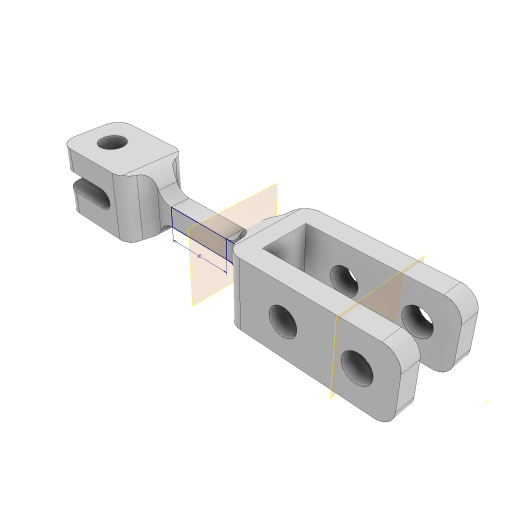
# Autodesk Inventor part: Acoplador
Saved by Autodesk Inventor 2023.5 (Build 275446020, 446B)
## iProperties
Created: 2025-07-10
Part Number: Acoplador
Material: Genérico
Document SubType Name: Modeling
Designer: jaime
Density: 1 g/cm^3
Appearance: Valor por defecto
Author: jaime
Autodesk Inventor part; units mm, degrees
ref_plane "YZ Plane" through (0, 0, 0) normal (1, 0, 0) x (0, 1, 0)
ref_plane "XZ Plane" through (0, 0, 0) normal (0, 1, 0) x (-1, 0, 0)
ref_plane "XY Plane" through (0, 0, 0) normal (0, 0, 1) x (1, 0, 0)
sketch "Boceto1" plane through (0, 0, 0) normal (0, 0, 1) x (1, 0, 0)
  circle A0 centre (0, 0) radius 2
  line L0 (0, 0) -> (10, 0)
  circle A1 centre (10, 0) radius 2
  line L1 (2, 0) -> (8, 0)
  line L2 (2, 0) -> (8, 0)
  line L3 (-5, -5) -> (15, -5)
  line L4 (15, -5) -> (15, 5)
  line L5 (15, 5) -> (-5, 5)
  line L6 (-5, -5) -> (15, 5) construction
  line L7 (15, -5) -> (-5, 5) construction
  line L8 (-5, 5) -> (-9, 5)
  line L9 (-9, 5) -> (-9, -5)
  line L10 (-9, -5) -> (-5, -5)
  point P0 (5, 0)
  dimension "d0" = 4
  dimension "d1" = 10
  dimension "d2" = 20
  dimension "d3" = 10
  dimension "d7" = 4
  constraints: 22 end point, 3 horizontal, 3 midpoint, 3 perpendicular, 2 coincident, 2 horizontal alignment, 2 point on line, 1 collinear, 1 parallel, 4 other
  measures "d1" distance of L0.start L0.end
  measures "d2" distance of L5.end L4.end
  measures "d3" distance of L4.end L3.end
  measures "d7" distance of L5.end L8.end
extrude "Extrusión1" add sketch "Boceto1" along normal blind 13
sketch "Boceto2" plane through (15, -5, 0) normal (1, 0, 0) x (0, 0, -1)
  line L0 (0, 10) -> (-13, 10) projected
  line L1 (-10, 0) -> (-3, 0)
  line L2 (-3, 0) -> (-3, 10)
  line L3 (-3, 10) -> (-10, 10)
  line L4 (-10, 10) -> (-10, 0)
  line L5 (-10, 0) -> (-3, 10) construction
  line L6 (-3, 0) -> (-10, 10) construction
  point P0 (0, 5)
  point P1 (-6.5, 5)
  dimension "d6" = 7
  constraints: 12 end point, 2 midpoint, 2 parallel, 1 horizontal, 1 perpendicular, 1 point on line
  measures "d6" distance of L3.end L2.end
extrude "Extrusión2" cut sketch "Boceto2" against normal blind 21
sketch "Boceto3" plane through (-9, -5, 0) normal (-1, 0, 0) x (0, 0, 1)
  line L0 (0, 0) -> (13, 0) projected
  line L1 (8, 10) -> (5, 10)
  line L2 (5, 10) -> (5, 0)
  line L3 (5, 0) -> (8, 0)
  line L4 (8, 0) -> (8, 10)
  line L5 (8, 10) -> (5, 0) construction
  line L6 (5, 10) -> (8, 0) construction
  point P0 (0, 5)
  point P1 (6.5, 5)
  dimension "d10" = 3
  constraints: 12 end point, 2 midpoint, 2 parallel, 1 horizontal, 1 perpendicular, 1 point on line
  measures "d10" distance of L3.end L2.end
extrude "Extrusión3" add sketch "Boceto3" along normal blind 55
sketch "Boceto4" plane through (-9, -5, 8) normal (0, 0, 1) x (1, 0, 0)
  line L0 (0, 10) -> (0, 0) projected
  line L1 (0, 5) -> (-48, 5)
  line L2 (-55, 10) -> (-55, 0) projected
  line L3 (-41, 3.5) -> (-55, 3.5)
  line L4 (-55, 3.5) -> (-55, 6.5)
  line L5 (-55, 6.5) -> (-41, 6.5)
  line L6 (-41, 6.5) -> (-41, 3.5)
  line L7 (-41, 3.5) -> (-55, 6.5) construction
  line L8 (-55, 3.5) -> (-41, 6.5) construction
  line L9 (-41, 3.5) -> (-41, 0)
  line L10 (0, 0) -> (-55, 0) projected
  line L11 (0, 10) -> (-55, 10) projected
  line L12 (-41, 6.5) -> (-55, 6.5)
  line L13 (-55, 6.5) -> (-55, 10)
  line L14 (-55, 10) -> (-41, 10)
  line L15 (-41, 10) -> (-41, 6.5)
  line L16 (-55, 3.5) -> (-41, 3.5)
  line L17 (-41, 3.5) -> (-41, 0)
  line L18 (-41, 0) -> (-55, 0)
  line L19 (-55, 0) -> (-55, 3.5)
  point P0 (9, 5)
  dimension "d13" = 48
  dimension "d14" = 3
  constraints: 32 end point, 6 parallel, 4 horizontal, 3 midpoint, 3 perpendicular, 2 point on line, 1 vertical
  measures "d13" distance of L1.start L1.end
  measures "d14" distance of L3.end L4.end
extrude "Extrusión4" cut sketch "Boceto4" against normal blind 55 contours L15 L5 L2 L11 | L10 L2 L3 L9
sketch "Boceto5" plane through (-64, 1.5, 8) normal (0, 1, 0) x (1, 0, 0)
  circle A0 centre (7, 1.5) radius 2
  line L0 (14, 6.5) -> (0, 6.5)
  line L1 (0, 6.5) -> (0, -3.5)
  line L2 (0, -3.5) -> (14, -3.5)
  line L3 (14, -3.5) -> (14, 6.5)
  line L4 (14, 6.5) -> (0, -3.5) construction
  line L5 (0, 6.5) -> (14, -3.5) construction
  point P0 (64, 8)
  dimension "d18" = 4
  dimension "d20" = 10
  constraints: 12 end point, 2 midpoint, 2 parallel, 1 centre point, 1 horizontal, 1 perpendicular
  measures "d18" diameter of A0
  measures "d20" distance of L1.end L0.end
extrude "Extrusión5" add sketch "Boceto5" against normal blind 3
sketch "Boceto6" plane through (-64, 1.5, 1.5) normal (0, 1, 0) x (1, 0, 0)
  arc A0 (8.3229, -3.5) -> (5.6771, -3.5) centre (7, -5) ccw projected
  circle A1 centre (7, -5) radius 2
  point P0 (64, 1.5)
  point P1 (5.6771, -3.5)
  point P2 (8.3229, -3.5)
  constraints: 1 centre point, 1 coincident
extrude "Extrusión6" cut sketch "Boceto6" against normal blind 3
sketch "Boceto7" plane through (-9, 5, 0) normal (0, 1, 0) x (1, 0, 0)
  line L0 (-41, -8) -> (-41, -11.5) projected
  line L1 (-41, -11.5) -> (-41, -10)
  line L2 (-39, -8) -> (-34.5905, -8)
  arc A0 (-39, -8) -> (-41, -10) centre (-39, -10) ccw
  line L3 (-41, -1.5) -> (-41, -5) projected
  line L4 (-38.5, -5) -> (-34.5905, -5)
  line L5 (0, -5) -> (-41, -5) projected
  line L6 (-41, -2.5) -> (-41, -1.5)
  arc A1 (-41, -2.5) -> (-38.5, -5) centre (-38.5, -2.5) ccw
  line L7 (-41, -2.5) -> (-41, -10)
  line L8 (-34.5905, -5) -> (-34.5905, -8)
  line L9 (0, -8) -> (-41, -8) projected
  point P0 (9, 0)
  point P1 (-38.5, -5)
  dimension "d25" = 2
  dimension "d26" = 2.5
  constraints: 12 end point, 5 point on line, 5 tangent, 4 point on circle, 3 perpendicular, 2 centre point, 1 collinear, 1 vertical
  measures "d25" radius of A0
  measures "d26" radius of A1
extrude "Extrusión7" add sketch "Boceto7" against normal blind 10 contours L9 A0 L0 | L3 A1 L5
sketch "Boceto8" plane through (-64, 1.5, 11.5) normal (0, 0, 1) x (1, 0, 0)
  line L0 (14, 3.5) -> (14, 0) projected
  line L1 (14, 3.5) -> (14, 3.5)
  line L2 (10.5, 0) -> (10.0047, 0)
  line L3 (0, 0) -> (14, 0) projected
  line L4 (0, -3) -> (14, -3) projected
  line L5 (10.0047, -3) -> (10.5, -3)
  line L6 (14, -3) -> (14, -6.5) projected
  line L7 (14, -6.5) -> (14, -6.5)
  line L8 (10.0047, -3) -> (10.0047, 0)
  line L9 (14, 2.5) -> (14, 3.5)
  arc A0 (14, -6.5) -> (10.5, -3) centre (10.5, -6.5) ccw
  arc A1 (10.5, 0) -> (14, 3.5) centre (10.5, 3.5) ccw
  line L10 (14, 2.5) -> (14, -6.5)
  point P0 (64, -1.5)
  point P1 (10.5, -3)
  dimension "d31" = 3.5
  dimension "d32" = 3.5
  constraints: 14 end point, 7 point on line, 4 point on circle, 4 tangent, 2 centre point, 2 collinear, 2 vertical, 1 perpendicular
  measures "d31" radius of A0
  measures "d32" radius of A1
extrude "Extrusión8" add sketch "Boceto8" against normal blind 10
sketch "Boceto9" plane through (-64, 1.5, 11.5) normal (0, 1, 0) x (1, 0, 0)
  line L0 (14, 0) -> (10.5, 0) projected
  line L1 (0, 10) -> (14, 10)
  line L2 (14, 10) -> (14, 0)
  line L3 (14, 0) -> (0, 0)
  line L4 (0, 0) -> (0, 10)
  circle A0 centre (7, 5) radius 2 projected
  circle A1 centre (7, 5) radius 2
  point P0 (64, 11.5)
  constraints: 8 end point, 2 parallel, 1 centre point, 1 coincident, 1 horizontal, 1 perpendicular
extrude "Extrusión9" add sketch "Boceto9" along normal blind 3.5
sketch "Boceto10" plane through (-64, -1.5, 1.5) normal (0, -1, 0) x (1, 0, 0)
  circle A0 centre (7, 5) radius 2 projected
  circle A1 centre (7, 5) radius 2
  line L0 (0, 10) -> (0, 0) projected
  line L1 (14, 0) -> (10.5, 0) projected
  line L2 (0, 10) -> (14, 10)
  line L3 (14, 10) -> (14, 0)
  line L4 (14, 0) -> (0, 0)
  line L5 (0, 0) -> (0, 10)
  point P0 (64, -1.5)
  constraints: 8 end point, 2 parallel, 1 centre point, 1 coincident, 1 horizontal, 1 perpendicular
extrude "Extrusión10" add sketch "Boceto10" along normal blind 3.5
sketch "Boceto11" plane through (-64, -5, 0) normal (-1, 0, 0) x (0, 0, 1)
  line L0 (11.5, 0) -> (11.5, 10) projected
  line L1 (1.5, 3.5) -> (11.5, 3.5)
  line L2 (11.5, 3.5) -> (11.5, 6.5)
  line L3 (11.5, 6.5) -> (1.5, 6.5)
  line L4 (1.5, 6.5) -> (1.5, 3.5)
  line L5 (1.5, 3.5) -> (11.5, 6.5) construction
  line L6 (11.5, 3.5) -> (1.5, 6.5) construction
  point P0 (0, 5)
  point P1 (6.5, 5)
  dimension "d39" = 3
  constraints: 12 end point, 2 midpoint, 2 parallel, 1 horizontal, 1 perpendicular, 1 point on line
  measures "d39" distance of L2.end L1.end
extrude "Extrusión11" cut sketch "Boceto11" against normal blind 11
fillet "Empalme1" radius 2.5 1 edges at (-50, 0, 1.5)
fillet "Empalme2" radius 2.5 1 edges at (-50, 0, 11.5)
fillet "Empalme3" radius 2.5 1 edges at (-9, 0, 5)
fillet "Empalme4" radius 2.5 1 edges at (-9, 0, 0)
fillet "Empalme5" radius 2.5 1 edges at (-9, 0, 8)
fillet "Empalme6" radius 2.5 1 edges at (-9, 0, 13)
sketch "Boceto12" plane through (-48, -5, 8) normal (0, 0, 1) x (1, 0, 0)
  line L0 (36.5, 10) -> (0, 10) projected
  line L1 (36.5, 10) -> (36.5, 0) projected
  line L2 (0, 10) -> (36.5, 10)
  line L3 (36.5, 10) -> (36.5, 9)
  line L4 (36.5, 0) -> (0, 0)
  line L5 (0, 9) -> (0, 10)
  line L6 (2.5, 3.5) -> (34, 3.5)
  line L7 (36.5, 3.5) -> (36.5, 6.5)
  line L8 (34, 6.5) -> (2.5, 6.5)
  line L9 (0, 6.5) -> (0, 3.5)
  line L10 (0, 3.5) -> (36.5, 6.5) construction
  line L11 (36.5, 3.5) -> (0, 6.5) construction
  arc A0 (0, 9) -> (2.5, 6.5) centre (2.5, 9) ccw
  arc A1 (34, 6.5) -> (36.5, 9) centre (34, 9) ccw
  line L12 (0, 0) -> (0, 10) projected
  line L13 (0, 1) -> (0, 0)
  line L14 (0, 0) -> (36.5, 0)
  arc A2 (2.5, 3.5) -> (0, 1) centre (2.5, 1) ccw
  line L15 (36.5, 1) -> (36.5, 0)
  arc A3 (36.5, 1) -> (34, 3.5) centre (34, 1) ccw
  line L16 (-4.3875, 10) -> (-4.3875, 0) projected
  line L17 (-4.3875, 6.5) -> (2.5, 6.5)
  line L18 (-4.3875, 10) -> (-4.3875, 6.5)
  point P0 (48, 5)
  point P1 (18.25, 5)
  dimension "d48" = 3
  dimension "d49" = 2.5
  dimension "d50" = 2.5
  dimension "d51" = 2.5
  dimension "d52" = 2.5
  constraints: 30 end point, 10 point on line, 8 point on circle, 8 tangent, 4 centre point, 4 parallel, 4 perpendicular, 2 collinear, 2 horizontal, 2 midpoint, 1 vertical
  measures "d48" distance of L7.end L7.start
  measures "d49" radius of A0
  measures "d50" radius of A1
  measures "d51" radius of A2
  measures "d52" radius of A3
extrude "Extrusión12" cut sketch "Boceto12" against normal blind 11 contours L1 A1 L8 A0 L5 L0 | L1 L4 L12 A2 L6 A3
fillet "Empalme7" radius 3.5 1 edges at (-11.5, 5, 6.5)
fillet "Empalme8" radius 3.5 1 edges at (-11.5, -5, 6.5)
fillet "Empalme9" radius 3.5 1 edges at (-48, 5, 6.4747)
fillet "Empalme10" radius 3.5 1 edges at (-48, -5, 6.4747)
fillet "Empalme11" radius 2.5 4 edges at (-64, 3.25, 11.5) (-64, -3.25, 11.5) (-64, 3.25, 1.5) (-64, -3.25, 1.5)
sketch "Boceto15" plane through (-50.9544, 5, 11.0485) normal (0, 1, 0) x (1, 0, 0)
  line L0 (-2.0456, 9.5485) -> (-2.0456, -0.4515) projected
  line L1 (-10.5456, 9.5485) -> (-2.0456, 9.5485) projected
  line L2 (-2.0456, -0.4515) -> (-8.0338, -0.4515)
  line L3 (-8.0338, -0.4515) -> (-8.0338, 9.5485)
  line L4 (-8.0338, 9.5485) -> (-2.0456, 9.5485)
  line L5 (-2.0456, 9.5485) -> (-2.0456, -0.4515)
  point P0 (50.9544, 11.0485)
  constraints: 8 end point, 2 parallel, 1 horizontal, 1 perpendicular, 1 point on line
extrude "Extrusión13" add sketch "Boceto15" against normal blind 10
sketch "Boceto16" plane through (-50.9544, 5, 11.0485) normal (0, 1, 0) x (1, 0, 0)
  line L0 (-13.0456, 7.0485) -> (-13.0456, 2.0485) projected
  line L1 (-13.0456, 4.5485) -> (-8.0456, 4.5485)
  circle A0 centre (-8.0456, 4.5485) radius 2
  point P0 (50.9544, 11.0485)
  dimension "d65" = 5
  dimension "d66" = 4
  constraints: 2 end point, 1 centre point, 1 coincident, 1 horizontal, 1 midpoint
  measures "d65" distance of L1.start L1.end
  measures "d66" diameter of A0
extrude "Extrusión14" cut sketch "Boceto16" against normal blind 10
sketch "Boceto17" plane through (-52.3875, -5, 11.5) normal (0, 0, 1) x (1, 0, 0)
  line L0 (-6.6007, 6.5) -> (-6.6007, 3.5) projected
  line L1 (-6.6007, 6.5) -> (-3.1007, 6.5)
  line L2 (-3.1007, 6.5) -> (-3.1007, 3.5)
  line L3 (-3.1007, 3.5) -> (-6.6007, 3.5)
  line L4 (-6.6007, 3.5) -> (-6.6007, 6.5)
  point P0 (52.3875, 5)
  dimension "d69" = 3.5
  dimension "d70" = 3
  constraints: 8 end point, 2 parallel, 1 horizontal, 1 perpendicular
  measures "d69" distance of L2.end L3.end
  measures "d70" distance of L1.end L2.end
extrude "Extrusión15" cut sketch "Boceto17" against normal blind 10
fillet "Empalme12" radius 2.5 4 edges at (15, 5, 11.5) (15, 5, 1.5) (15, -5, 1.5) (15, -5, 11.5)
sketch "Boceto18" plane through (-45.5, -1.5, 8) normal (0, 0, 1) x (1, 0, 0)
  line L0 (0, 3) -> (31.5, 3)
  line L1 (31.5, 3) -> (31.5, 0)
  line L2 (31.5, 0) -> (0, 0)
  line L3 (0, 0) -> (0, 3)
  line L4 (0, 3) -> (31.5, 3) projected
  line L5 (31.5, 0) -> (0, 0) projected
  line L6 (0, 3) -> (10, 3)
  line L7 (10, 3) -> (10, 0)
  line L8 (10, 0) -> (0, 0)
  line L9 (0, 0) -> (0, 3)
  point P0 (45.5, 1.5)
  dimension "d74" = 10
  constraints: 16 end point, 4 parallel, 2 horizontal, 2 perpendicular, 1 point on line
  measures "d74" distance of L7.end L8.end
ref_plane "Plano de trabajo1" through (-35.5, 1.5, 8) normal (1, 0, 0) x (0, -1, 0)
ref_plane "Plano de trabajo2" through (-14, 1.5, 8) normal (1, 0, 0) x (0, -1, 0)
split body "Dividir1" result two bodies by plane through (-35.5, 1.5, 8) normal (1, 0, 0) first body at (2.0803, 3.9951, 12.5)
split "Dividir2" plane through (-14, 1.5, 8) removes the side toward (-1, 0, 0) bodies 2
move or copy body "Desplazar cuerpo1" bodies to move or copy 2 copy no translate (-21.5, 0, 0)
combine bodies "Combinar1" operation type add bodies to combine 2 3
sketch "Boceto19" plane through (-61.5, -5, 11.5) normal (0, 0, 1) x (1, 0, 0)
  line L0 (6.0119, 6.5) -> (6.0119, 3.5) projected
  line L1 (6.0119, 5) -> (7.8119, 5)
  ellipse E0 centre (6.0119, 5) end of major axis (6.0119, 6.5) minor radius 1.8053
  point P0 (61.5, 5)
  dimension "d80" = 1.8
  constraints: 2 end point, 1 coincident, 1 horizontal, 1 midpoint, 1 vertical, 3 other
  measures "d80" distance of L1.start L1.end
extrude "Extrusión16" cut sketch "Boceto19" against normal blind 20 contours E0 L0 picked at (6.7383, 4.2134) bodies 2
